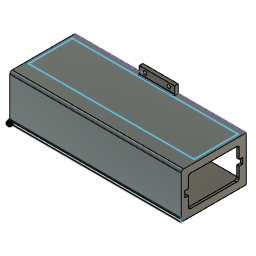
Battery holder v6 (Autodesk Fusion 360 design; units mm, degrees)
Autodesk Fusion 360 part; units mm, degrees
sketch "Sketch1" plane through (0, 0, 0) normal (0, 0, 1) x (1, 0, 0)
  line L0 (70, 25) -> (-70, 25)
  line L1 (-70, 25) -> (-70, -25)
  line L2 (-70, -25) -> (70, -25)
  line L3 (70, -25) -> (70, 25)
  line L4 (70, 25) -> (-70, -25) construction
  line L5 (-70, 25) -> (70, -25) construction
  dimension "d1" = 140
  dimension "d2" = 50
  constraint horizontal L0
  constraint perpendicular L0 L1
  constraint parallel L0 L2
  constraint parallel L1 L3
  constraint coincident L4 origin
  constraint coincident L5 origin
  measures "d1" distance of L1.end L2.end
  measures "d2" distance of L0.end L1.end
extrude "Extrude1" add sketch "Sketch1" along normal blind 30
sketch "Sketch2" plane through (0, 0, 0) normal (0, 0, -1) x (1, 0, 0)
  line L0 (70, -25) -> (70, 25)
  line L1 (70, 25) -> (-70, 25)
  line L2 (-70, 25) -> (-70, -25)
  line L3 (-70, -25) -> (70, -25)
  line L4 (-72.5, 27.5) -> (72.5, 27.5)
  line L5 (72.5, 27.5) -> (72.5, -27.5)
  line L6 (72.5, -27.5) -> (-72.5, -27.5)
  line L7 (-72.5, -27.5) -> (-72.5, 27.5)
  line L8 (-72.5, 27.5) -> (72.5, -27.5) construction
  line L9 (72.5, 27.5) -> (-72.5, -27.5) construction
  dimension "d5" = 145
  dimension "d6" = 55
  constraint horizontal L4
  constraint perpendicular L4 L5
  constraint parallel L4 L6
  constraint parallel L5 L7
  constraint coincident L8 origin
  constraint coincident L9 origin
  measures "d5" distance of L5.end L6.end
  measures "d6" distance of L4.end L5.end
extrude "Extrude2" cut 1 faces at (-23.3333, 8.3333, 30) along direction (0, 0, -1) blind 30
extrude "Extrude3" add sketch "Sketch2" against normal blind 35
sketch "Sketch3" plane through (0, 0, 0) normal (0, 0, -1) x (1, 0, 0)
  line L0 (70, -25) -> (-70, -25)
  line L1 (-70, -25) -> (-70, 25)
  line L2 (-70, 25) -> (70, 25)
  line L3 (70, 25) -> (70, -25)
  line L4 (-72.5, -27.5) -> (72.5, -27.5)
  line L5 (72.5, -27.5) -> (72.5, 27.5)
  line L6 (72.5, 27.5) -> (-72.5, 27.5)
  line L7 (-72.5, 27.5) -> (-72.5, -27.5)
  line L8 (72.5, -27.5) -> (-72.5, -27.5)
  line L9 (-72.5, -27.5) -> (-72.5, 27.5)
  line L10 (-72.5, 27.5) -> (72.5, 27.5)
  line L11 (72.5, 27.5) -> (72.5, -27.5)
  constraint horizontal L8
  constraint vertical L9
  constraint horizontal L10
  constraint vertical L11
  constraint coincident L6.end L7.start
  constraint coincident L4.end L5.start
extrude "Extrude4" add sketch "Sketch3" along normal blind 3 contours L0 L1 L2 L3 | L4 L5 L6 L7 L8 L9 L10 L11
sketch "Sketch4" plane through (-72.5, 0, 0) normal (-1, 0, 0) x (0, -1, 0)
  line L0 (27.5, -3) -> (27.5, 35)
  line L1 (27.5, 35) -> (-27.5, 35)
  line L2 (-27.5, 35) -> (-27.5, -3)
  line L3 (-27.5, -3) -> (27.5, -3)
  line L4 (21.5, 3) -> (21.5, 29)
  line L5 (21.5, 29) -> (-21.5, 29)
  line L6 (-21.5, 29) -> (-21.5, 3)
  line L7 (-21.5, 3) -> (21.5, 3)
  dimension "d13" = -6
extrude "Extrude5" cut sketch "Sketch4" against normal blind 240 contours L4 L5 L6 L7
fillet "Fillet1" radius 2 2 edges at (0, 25, 0) (0, -25, 0)
fillet "Fillet2" radius 2 8 edges at (71.25, -21.5, 29) (71.25, -21.5, 3) (71.25, 21.5, 3) (71.25, 21.5, 29) (-71.25, -21.5, 29) (-71.25, 21.5, 29) (-71.25, 21.5, 3) (-71.25, -21.5, 3)
sketch "Sketch5" plane through (-72.5, 0, 0) normal (-1, 0, 0) x (0, -1, 0)
  line L0 (21.5, 27) -> (21.5, 5)
  arc A0 (19.5, 3) -> (21.5, 5) centre (19.5, 5) ccw
  line L1 (19.5, 3) -> (-19.5, 3)
  arc A1 (-21.5, 5) -> (-19.5, 3) centre (-19.5, 5) ccw
  line L2 (-21.5, 5) -> (-21.5, 27)
  arc A2 (-19.5, 29) -> (-21.5, 27) centre (-19.5, 27) ccw
  line L3 (-19.5, 29) -> (19.5, 29)
  arc A3 (21.5, 27) -> (19.5, 29) centre (19.5, 27) ccw
  line L4 (27.5, -3) -> (27.5, 35)
  line L5 (27.5, 35) -> (-27.5, 35)
  line L6 (-27.5, 35) -> (-27.5, -3)
  line L7 (-27.5, -3) -> (27.5, -3)
  line L8 (-24.5, 18.5) -> (24.5, 18.5)
  line L9 (24.5, 18.5) -> (24.5, 13.5)
  line L10 (24.5, 13.5) -> (-24.5, 13.5)
  line L11 (-24.5, 13.5) -> (-24.5, 18.5)
  line L12 (-24.5, 18.5) -> (24.5, 13.5) construction
  line L13 (24.5, 18.5) -> (-24.5, 13.5) construction
  point P0 (0, 16)
  dimension "d20" = 49
  dimension "d21" = 5
  constraint horizontal L8
  constraint perpendicular L8 L9
  constraint parallel L8 L10
  constraint parallel L9 L11
  constraint coincident L12 P0
  constraint coincident L13 P0
  measures "d20" distance of L9.end L10.end
  measures "d21" distance of L8.end L9.end
extrude "Extrude6" cut sketch "Sketch5" against normal blind 190 contours L0 L8 L9 L10 | L2 L8 L10 L11
fillet "Fillet3" radius 1 8 edges at (-71.25, -24.5, 18.5) (-71.25, -21.5, 18.5) (-71.25, -21.5, 13.5) (-71.25, -24.5, 13.5) (-71.25, 21.5, 18.5) (-71.25, 21.5, 13.5) (-71.25, 24.5, 13.5) (-71.25, 24.5, 18.5)
sketch "Sketch6" plane through (70, 0, 0) normal (-1, 0, 0) x (0, -1, 0)
  line L0 (-24.5, 18.5) -> (-21.5, 18.5)
  line L1 (-21.5, 18.5) -> (-21.5, 27)
  arc A0 (-19.5, 29) -> (-21.5, 27) centre (-19.5, 27) ccw
  line L2 (-19.5, 29) -> (19.5, 29)
  arc A1 (21.5, 27) -> (19.5, 29) centre (19.5, 27) ccw
  line L3 (21.5, 27) -> (21.5, 18.5)
  line L4 (21.5, 18.5) -> (24.5, 18.5)
  line L5 (24.5, 18.5) -> (24.5, 13.5)
  line L6 (24.5, 13.5) -> (21.5, 13.5)
  line L7 (21.5, 13.5) -> (21.5, 5)
  arc A2 (19.5, 3) -> (21.5, 5) centre (19.5, 5) ccw
  line L8 (19.5, 3) -> (-19.5, 3)
  arc A3 (-21.5, 5) -> (-19.5, 3) centre (-19.5, 5) ccw
  line L9 (-21.5, 5) -> (-21.5, 13.5)
  line L10 (-21.5, 13.5) -> (-24.5, 13.5)
  line L11 (-24.5, 13.5) -> (-24.5, 18.5)
  arc A4 (23, 0) -> (25, 2) centre (23, 2) ccw
  line L12 (25, 2) -> (25, 35)
  line L13 (25, 35) -> (-25, 35)
  line L14 (-25, 35) -> (-25, 2)
  arc A5 (-25, 2) -> (-23, 0) centre (-23, 2) ccw
  line L15 (-23, 0) -> (23, 0)
  line L16 (25, 35) -> (18.3622, 35)
  line L17 (18.3622, 35) -> (18.3622, 33)
  line L18 (18.3622, 33) -> (25, 33)
  line L19 (25, 33) -> (25, 35)
  constraint horizontal L16
  constraint vertical L17
  constraint horizontal L18
  constraint vertical L19
  constraint coincident L12.end L13.start
extrude "Extrude7" add sketch "Sketch6" along normal blind 140 contours L12 L13 L16 L17 L18 L19
sketch "Sketch7" plane through (0, 0, 0) normal (0, 0, 1) x (-1, 0, 0)
  line L0 (70, 23) -> (-70, 23)
  line L1 (-70, 23) -> (-70, -23)
  line L2 (-70, -23) -> (70, -23)
  line L3 (70, -23) -> (70, 23)
  line L4 (0, 0) -> (0, -27.5) construction
  line L5 (0, 0) -> (0, 27.5) construction
  circle A0 centre (-5, 0) radius 1.5
  circle A1 centre (5, 0) radius 1.5
  circle A2 centre (0, -13) radius 1.5
  circle A3 centre (0, 11) radius 1.5
  dimension "d28" = 3
  dimension "d29" = 3
  dimension "d30" = 3
  dimension "d31" = 3
  constraint coincident L4.start L5.start
  constraint perpendicular L2 L4
  constraint parallel L4 L5
  constraint coincident L4 A2.centre
  measures "d28" diameter of A0
  measures "d29" diameter of A1
  measures "d30" diameter of A2
  measures "d31" diameter of A3
sketch "Sketch9" plane through (0, -27.5, 0) normal (0, -1, 0) x (1, 0, 0)
  line L0 (72.5, -3) -> (72.5, 35)
  line L1 (72.5, 35) -> (-72.5, 35)
  line L2 (-72.5, 35) -> (-72.5, -3)
  line L3 (-72.5, -3) -> (72.5, -3)
  line L4 (-72.5, -3) -> (72.5, -3)
  line L5 (72.5, -3) -> (72.5, 0)
  line L6 (72.5, 0) -> (-72.5, 0)
  line L7 (-72.5, 0) -> (-72.5, -3)
  dimension "d40" = 3
  constraint horizontal L4
  constraint vertical L5
  constraint horizontal L6
  constraint vertical L7
  constraint coincident L2.end L3.start
  measures "d40" distance of L2.end L6.end
extrude "Extrude9" add 1 faces at (23.3333, -18.3622, 34.3333) along direction (0, 1, 0) up to surface (43.3622 mm away)
sketch "Sketch10" plane through (0, 27.5, 0) normal (0, 1, 0) x (-1, 0, 0)
  line L0 (72.5, -3) -> (72.5, 35)
  line L1 (72.5, 35) -> (-72.5, 35)
  line L2 (-72.5, 35) -> (-72.5, -3)
  line L3 (-72.5, -3) -> (72.5, -3)
  line L4 (70.5, -1) -> (70.5, 33)
  line L5 (70.5, 33) -> (-70.5, 33)
  line L6 (-70.5, 33) -> (-70.5, -1)
  line L7 (-70.5, -1) -> (70.5, -1)
  dimension "d43" = -2
extrude "Extrude10" cut sketch "Sketch10" against normal blind 53 contours L4 L5 L6 L7
fillet "Fillet6" radius 2 2 edges at (0, -25.5, 33) (0, -25.5, -1)
sketch "Sketch11" plane through (0, -27.5, 0) normal (0, -1, 0) x (1, 0, 0)
  line L0 (15, -10) -> (-15, -10)
  line L1 (-15, -10) -> (-15, 42)
  line L2 (-15, 42) -> (15, 42)
  line L3 (15, 42) -> (15, -10)
  line L4 (15, -10) -> (-15, 42) construction
  line L5 (-15, -10) -> (15, 42) construction
  line L6 (15, -10) -> (-15, -10)
  line L7 (-15, -10) -> (-15, -3)
  line L8 (-15, -3) -> (15, -3)
  line L9 (15, -3) -> (15, -10)
  line L10 (-15, 35) -> (15, 35)
  line L11 (15, 35) -> (15, 42)
  line L12 (15, 42) -> (-15, 42)
  line L13 (-15, 42) -> (-15, 35)
  point P0 (0, 16)
  constraint horizontal L0
  constraint perpendicular L0 L1
  constraint parallel L0 L2
  constraint parallel L1 L3
  constraint coincident L4 P0
  constraint coincident L5 P0
  constraint horizontal L6
  constraint vertical L7
  constraint horizontal L8
  constraint vertical L9
  constraint coincident L1 L7.end
  constraint horizontal L10
  constraint vertical L11
  constraint horizontal L12
  constraint vertical L13
  constraint coincident L1 L10.start
extrude "Extrude11" add sketch "Sketch11" against normal blind 3 from surface at -52 contours L0 L1 L3 L6 L7 L8 L9 | L1 L2 L3 L10 L11 L12 L13
sketch "Sketch12" plane through (0, 27.5, 0) normal (0, 1, 0) x (-1, 0, 0)
  line L0 (15, 35) -> (15, 42)
  line L1 (15, 42) -> (-15, 42)
  line L2 (-15, 42) -> (-15, 35)
  circle A0 centre (0, 39) radius 1.5
  circle A1 centre (0, -7) radius 1.5
  circle A2 centre (10, -7) radius 1.5
  circle A3 centre (-10, -7) radius 1.5
  circle A4 centre (-10, 39) radius 1.5
  circle A5 centre (10, 39) radius 1.5
  line L3 (70.5, 33) -> (70.5, -1)
  line L4 (70.5, -1) -> (-70.5, -1)
  line L5 (-70.5, -1) -> (-70.5, 33)
  line L6 (-70.5, 33) -> (70.5, 33)
  line L7 (-72.5, 35) -> (-72.5, -3)
  line L8 (-15, -3) -> (-15, -10)
  line L9 (-15, -10) -> (15, -10)
  line L10 (15, -10) -> (15, -3)
  line L11 (72.5, -3) -> (72.5, 35)
  line L12 (72.5, 35) -> (15, 35)
  line L13 (-15, 35) -> (-72.5, 35)
  line L14 (-72.5, -3) -> (-15, -3)
  line L15 (15, -3) -> (72.5, -3)
  dimension "d54" = 3
  dimension "d55" = 3
  dimension "d56" = 3
  dimension "d57" = 3
  dimension "d58" = 3
  dimension "d59" = 3
  measures "d54" diameter of A0
  measures "d55" diameter of A1
  measures "d56" diameter of A2
  measures "d57" diameter of A3
  measures "d58" diameter of A4
  measures "d59" diameter of A5
extrude "Extrude12" cut sketch "Sketch12" against normal blind 6 contours A2 | A3 | A4 | A5
sketch "Sketch13" plane through (0, 0, 35) normal (0, 0, 1) x (-1, 0, 0)
  line L0 (72.5, -27.5) -> (72.5, 27.5)
  line L1 (72.5, 27.5) -> (-72.5, 27.5)
  line L2 (-72.5, 27.5) -> (-72.5, -27.5)
  line L3 (-15, -27.5) -> (-15, -24.5)
  line L4 (-15, -24.5) -> (15, -24.5)
  line L5 (15, -24.5) -> (15, -27.5)
  line L6 (70, -22.984) -> (-70, -22.984)
  line L7 (-70, -22.984) -> (-70, 14)
  line L8 (-70, 14) -> (70, 14)
  line L9 (70, 14) -> (70, -22.984)
  line L10 (15, -27.5) -> (72.5, -27.5)
  line L11 (-72.5, -27.5) -> (-15, -27.5)
  constraint horizontal L6
  constraint vertical L7
  constraint horizontal L8
  constraint vertical L9
fillet "Fillet8" radius 2 2 edges at (0, -27.5, -3) (0, -27.5, 35)
fillet "Fillet9" radius 1 1 edges at (0, 24.5, -3)
fillet "Fillet10" radius 1 1 edges at (0, 24.5, 35)
